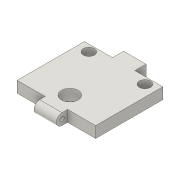
# Autodesk Inventor part: Deckel
Saved by Autodesk Inventor 2018.3 (Build 223284000, 284)
## iProperties
Created: 2019-11-28
Material: Stahl, unlegiert
Document SubType Name: Modeling
Designer: dirkb
Density: 7.85 g/cm^3
Appearance: Stahl
Description: Deckel
Werkstoff: S235JRC+C
Author: dirkb
Autodesk Inventor part; units mm, degrees
ref_plane "YZ Plane" through (0, 0, 0) normal (1, 0, 0) x (0, 1, 0)
ref_plane "XZ Plane" through (0, 0, 0) normal (0, 1, 0) x (-1, 0, 0)
ref_plane "XY Plane" through (0, 0, 0) normal (0, 0, 1) x (1, 0, 0)
sketch "Skizze_Grundkörper" plane through (0, 0, 0) normal (0, 0, 1) x (1, 0, 0)
  line L0 (-49, 0) -> (49, 0) projected
  line L1 (0, -56) -> (0, 56) projected
  line L2 (35, -40) -> (-35, -40)
  line L3 (-35, -40) -> (-35, 40)
  line L4 (-35, 40) -> (35, 40)
  line L5 (35, 40) -> (35, -40)
  line L6 (35, -40) -> (-35, 40) construction
  line L7 (-35, -40) -> (35, 40) construction
  point P0 (0, 0)
  dimension "Breite" = 70
  dimension "Länge" = 80
  constraints: 12 end point, 2 midpoint, 2 parallel, 1 horizontal, 1 perpendicular
  measures "Breite" distance of L3.end L4.end
  measures "Länge" distance of L4.end L2.start
extrude "Grundkörper" add sketch "Skizze_Grundkörper" along normal mid plane 10
sketch "Skizze_Ausnehmung" plane through (0, 0, 5) normal (0, 0, 1) x (1, 0, 0)
  line L0 (-49, 0) -> (49, 0) projected
  line L1 (0, -56) -> (0, 56) projected
  line L2 (-35, -40) -> (35, -40) projected
  line L3 (35, -40) -> (35, 40) projected
  line L4 (35, 40) -> (-35, 40) projected
  line L5 (-35, 40) -> (-35, -40) projected
  line L6 (-35, 40) -> (-10, 40)
  line L7 (-10, 40) -> (-10, 30)
  line L8 (-10, 30) -> (-35, 30)
  line L9 (-35, 30) -> (-35, 40)
  line L10 (35, 40) -> (-35, 40) projected
  line L11 (35, 40) -> (10, 40)
  line L12 (10, 40) -> (10, 30)
  line L13 (10, 30) -> (35, 30)
  line L14 (35, 30) -> (35, 40)
  line L15 (35, -40) -> (10, -40)
  line L16 (10, -40) -> (10, -30)
  line L17 (10, -30) -> (35, -30)
  line L18 (35, -30) -> (35, -40)
  line L19 (-35, 40) -> (-35, -40) projected
  line L20 (-35, -40) -> (-10, -40)
  line L21 (-10, -40) -> (-10, -30)
  line L22 (-10, -30) -> (-35, -30)
  line L23 (-35, -30) -> (-35, -40)
  point P0 (0, 0)
  dimension "d4" = 20
  dimension "d5" = 10
  constraints: 32 end point, 8 parallel, 4 horizontal, 4 perpendicular, 3 collinear, 3 other
  measures "d4" distance between parallel lines of L12 L7
  measures "d5" distance of L11.end L12.end
extrude "Ausnehmung" cut sketch "Skizze_Ausnehmung" against normal through all contours L5 L4 L7 L8 | L22 L21 L2 L5 | L3 L2 L16 L17 | L13 L12 L4 L3
full round fillet "Rundung1" first side at (-26.6667, 10, 5) centre faces at (-3.3333, -40, -1.6667) second side at (26.6667, -10, -5)
hole "Bohrung_4_mm" at (10, -35, 0) direction (-1, 0, 0) diameter 4 end through all
sketch "Skizze_15_mm" plane through (0, 0, 5) normal (0, 0, 1) x (1, 0, 0)
  line L0 (-49, 0) -> (49, 0) projected
  line L1 (0, -56) -> (0, 56) projected
  line L2 (10, -35) -> (-10, -35) projected
  line L3 (10, -35) -> (10, -30) projected
  line L4 (10, -30) -> (35, -30) projected
  line L5 (35, -30) -> (35, 30) projected
  line L6 (35, 30) -> (10, 30) projected
  line L7 (10, 30) -> (10, 40) projected
  line L8 (10, 40) -> (-10, 40) projected
  line L9 (-10, 40) -> (-10, 30) projected
  line L10 (-10, 30) -> (-35, 30) projected
  line L11 (-35, 30) -> (-35, -30) projected
  line L12 (-35, -30) -> (-10, -30) projected
  line L13 (-10, -30) -> (-10, -35) projected
  point P0 (0, 0)
  point P1 (0, -18)
  dimension "d17" = 58
  constraints: 1 point on line
  measures "d17" distance from line of point (0, -18) L8
hole "Bohrung_15_mm" at (0, -18, 5) direction (0, 0, -1) diameter 15 end through all
sketch "Skizze_Bohrung_10_mm" plane through (0, 0, 5) normal (0, 0, 1) x (1, 0, 0)
  line L0 (-49, 0) -> (49, 0) projected
  line L1 (0, -56) -> (0, 56) projected
  circle A0 centre (0, -18) radius 7.5 projected
  line L2 (10, -35) -> (-10, -35) projected
  line L3 (10, -35) -> (10, -30) projected
  line L4 (10, -30) -> (35, -30) projected
  line L5 (35, -30) -> (35, 30) projected
  line L6 (35, 30) -> (10, 30) projected
  line L7 (10, 30) -> (10, 40) projected
  line L8 (10, 40) -> (-10, 40) projected
  line L9 (-10, 40) -> (-10, 30) projected
  line L10 (-10, 30) -> (-35, 30) projected
  line L11 (-35, 30) -> (-35, -30) projected
  line L12 (-35, -30) -> (-10, -30) projected
  line L13 (-10, -30) -> (-10, -35) projected
  point P0 (0, 0)
  point P1 (-25, 24)
  point P2 (25, 24)
  dimension "d25" = 50
  dimension "d26" = 16
  constraints: 1 symmetric about line
  measures "d25" distance of point (25, 24) point (-25, 24)
  measures "d26" distance from line of L8 point (25, 24)
hole "Bohrung_10_mm" at (-25, 24, 5) at (25, 24, 5) direction (0, 0, -1) diameter 10 end through all
sketch "Skizze5" plane through (-10, 40, -5) normal (0, 1, 0) x (1, 0, 0)
  point P0 (10, -5)
  point P1 (10, -5)
  constraints: 1 coincident
hole "Bohrung_4_mm unten" at (0, 40, 0) direction (0, -1, 0) diameter 4 depth 10 tip angle 118
